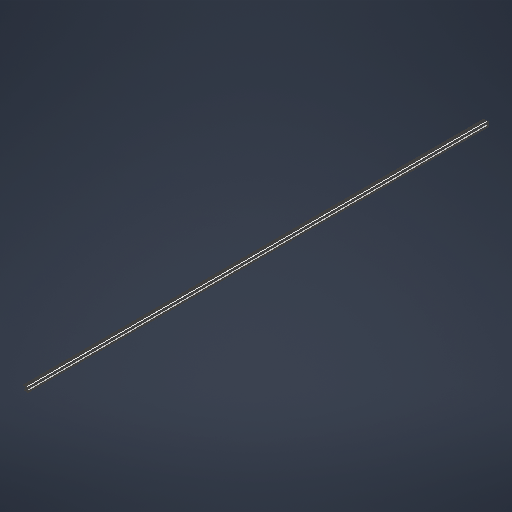
# Autodesk Inventor part: SP40-07 INVERSOR CENTRAL
Saved by Autodesk Inventor 2025 (Build 290162000, 162)
## iProperties
Created: 2026-01-24
Part Number: SP40-07 INVERSOR CENTRAL
Material: Aluminio
Document SubType Name: Modeling
Designer: ROLANDO
Density: 2.7 g/cm^3
Appearance: Satinado
Author: ROLANDO
Autodesk Inventor part; units mm, degrees
ref_plane "YZ Plane" through (0, 0, 0) normal (1, 0, 0) x (0, 1, 0)
ref_plane "XZ Plane" through (0, 0, 0) normal (0, 1, 0) x (-1, 0, 0)
ref_plane "XY Plane" through (0, 0, 0) normal (0, 0, 1) x (1, 0, 0)
sketch "Boceto1" plane through (0, 0, 0) normal (0, 0, 1) x (1, 0, 0)
  line L0 (8.6921, 12.0599) -> (8.6921, 49.4931)
  line L1 (8.6921, 10.6599) -> (-18.8079, 10.6599)
  line L2 (8.6921, 6.5599) -> (8.6921, 10.6599)
  line L3 (8.6921, 6.5599) -> (12.5921, 6.5599)
  line L4 (13.9921, 7.9599) -> (10.0921, 7.9599)
  line L5 (12.5921, 6.5599) -> (12.5921, 4.1599)
  line L6 (12.5921, 4.1599) -> (13.9921, 4.1599)
  line L7 (13.9921, 4.1599) -> (13.9921, 7.9599)
  line L8 (-13.0079, 12.0599) -> (-13.0079, 14.5599)
  line L9 (-13.0079, 14.5599) -> (-14.4079, 14.5599)
  line L10 (-14.4079, 14.5599) -> (-14.4079, 12.0599)
  line L11 (-8.6079, 12.0599) -> (-8.6079, 13.1599)
  line L12 (-8.6079, 14.5599) -> (-10.0079, 14.5599)
  line L13 (-10.0079, 14.5599) -> (-10.0079, 12.0599)
  line L14 (-7.2079, 14.1599) -> (-7.2079, 29.9599)
  line L15 (-8.6079, 29.5599) -> (-8.6079, 14.5599)
  line L16 (-17.4079, 12.0599) -> (-14.4079, 12.0599)
  line L17 (-17.4079, 12.0599) -> (-17.4079, 14.0599)
  line L18 (-18.8079, 12.9499) -> (-18.8079, 10.6599)
  line L19 (-17.4079, 14.0599) -> (-18.0102, 14.0599)
  line L20 (-18.0102, 14.0599) -> (-18.8079, 12.9499)
  line L21 (-8.6079, 29.5599) -> (-10.0079, 29.5599)
  line L22 (-10.0079, 29.5599) -> (-10.0079, 32.0599)
  line L23 (-8.6079, 33.4599) -> (-8.6079, 30.9599)
  line L24 (-18.8079, 29.4699) -> (-18.8079, 33.4599)
  line L25 (-14.4079, 32.0599) -> (-14.4079, 29.5599)
  line L26 (-14.4079, 29.5599) -> (-13.0079, 29.5599)
  line L27 (-13.0079, 29.5599) -> (-13.0079, 32.0599)
  line L28 (-10.0079, 32.0599) -> (-13.0079, 32.0599)
  line L29 (-14.4079, 32.0599) -> (-17.4079, 32.0599)
  line L30 (-17.4079, 32.0599) -> (-17.4079, 28.2599)
  line L31 (-17.4079, 28.2599) -> (-18.0191, 28.2599)
  line L32 (-13.0079, 33.4599) -> (-13.0079, 49.4999)
  line L33 (-14.4079, 49.4999) -> (-14.4079, 33.4599)
  line L34 (-18.8079, 33.4599) -> (-14.4079, 33.4599)
  line L35 (-13.0079, 33.4599) -> (-8.6079, 33.4599)
  line L36 (-13.0079, 49.4999) -> (-10.3179, 49.4999)
  line L37 (-10.3179, 49.4999) -> (-9.746, 50.1047)
  line L38 (-14.4079, 49.4999) -> (-17.0979, 49.4999)
  line L39 (-17.0979, 49.4999) -> (-17.5485, 49.9765)
  line L40 (-9.746, 50.1047) -> (8.6921, 49.4931)
  line L41 (-17.5485, 49.9765) -> (-27.9079, 49.669)
  line L42 (-27.9079, 49.669) -> (-27.9079, 45.6999)
  line L43 (-29.3079, 47.0999) -> (-29.3079, 49.4999)
  line L44 (-37.2079, 50.7936) -> (-37.2079, 45.6999)
  line L45 (-35.8079, 47.0999) -> (-35.8079, 49.4999)
  line L46 (-11.3879, 51.5599) -> (19.4921, 50.5356)
  line L47 (-11.3879, 51.5599) -> (-37.2079, 50.7936)
  line L48 (-8.6079, 30.9599) -> (-8.2079, 30.9599)
  line L49 (-8.6079, 13.1599) -> (-8.2079, 13.1599)
  line L50 (16.9921, 43.5999) -> (19.4921, 43.5999)
  line L51 (19.4921, 43.5999) -> (19.4921, 50.5356)
  line L52 (10.0921, 49.4466) -> (10.0921, 7.9599)
  line L53 (10.0921, 49.4466) -> (18.0921, 49.1812)
  line L54 (18.0921, 44.9999) -> (18.0921, 49.1812)
  line L55 (16.4921, 44.0999) -> (16.4921, 44.4999)
  line L56 (16.9921, 44.9999) -> (18.0921, 44.9999)
  line L57 (-13.0079, 12.0599) -> (-10.0079, 12.0599)
  line L58 (-8.6079, 12.0599) -> (8.6921, 12.0599)
  line L59 (-18.8079, 29.4699) -> (-18.0191, 28.2599)
  line L60 (-35.8079, 49.4999) -> (-29.3079, 49.4999)
  line L61 (-35.8079, 47.0999) -> (-34.5579, 47.0999)
  line L62 (-34.5579, 47.0999) -> (-34.5579, 46.3941)
  line L63 (-34.5579, 46.3941) -> (-35.5679, 45.6999)
  line L64 (-35.5679, 45.6999) -> (-37.2079, 45.6999)
  line L65 (-29.3079, 47.0999) -> (-30.5579, 47.0999)
  line L66 (-30.5579, 47.0999) -> (-30.5579, 46.3941)
  line L67 (-30.5579, 46.3941) -> (-29.5479, 45.6999)
  line L68 (-29.5479, 45.6999) -> (-27.9079, 45.6999)
  arc A0 (-7.2079, 29.9599) -> (-8.2079, 30.9599) centre (-8.2079, 29.9599) ccw
  arc A1 (-8.2079, 13.1599) -> (-7.2079, 14.1599) centre (-8.2079, 14.1599) ccw
  arc A2 (16.9921, 44.9999) -> (16.4921, 44.4999) centre (16.9921, 44.4999) ccw
  arc A3 (16.4921, 44.0999) -> (16.9921, 43.5999) centre (16.9921, 44.0999) ccw
  point P0 (0, 0)
  point P1 (-7.2079, 30.9599)
  point P2 (-7.2079, 13.1599)
  point P3 (16.4921, 43.5999)
  point P4 (16.4921, 44.9999)
  point P5 (-32.5579, 49.4999)
  dimension "d0" = 3.02
  dimension "d1" = 24.5
  dimension "d2" = 1.4
  dimension "d3" = 1.4
  dimension "d4" = 1.4
  dimension "d5" = 1.4
  dimension "d7" = 1.4
  dimension "d8" = 1.4
  dimension "d9" = 1.4
  dimension "d10" = 1.4
  dimension "d11" = 1.4
  dimension "d12" = 1.4
  dimension "d13" = 1.4
  dimension "d14" = 1.4
  dimension "d15" = 1.4
  dimension "d16" = 1.4
  dimension "d17" = 1.4
  dimension "d23" = 1.4
  dimension "d26" = 3
  dimension "d27" = 39.44
  dimension "d31" = 7.9
  dimension "d32" = 2.4
  dimension "d34" = 2.5
  dimension "d35" = 2.5
  dimension "d36" = 3
  dimension "d37" = 3
  dimension "d38" = 3
  dimension "d39" = 3
  dimension "d42" = 4.09
  dimension "d43" = 2.69
  dimension "d44" = 15
  dimension "d45" = 20
  dimension "d47" = 2
  dimension "d48" = 1.11
  dimension "d51" = 1.21
  dimension "d52" = 35.7
  dimension "d53" = 33.1
  dimension "d55" = 32.8
  dimension "d56" = 14.2
  dimension "d58" = 15.9
  dimension "d65" = 1.4
  dimension "d68" = 46.6
  dimension "d69" = 46.6
  dimension "d70" = 2.06
  dimension "d73" = 91.7
  dimension "d74" = 91.9
  dimension "d77" = 1.4
  dimension "d84" = 1.4
  dimension "d87" = 6.5
  dimension "d88" = 9.3
  dimension "d89" = 1.4
  dimension "d90" = 1.4
  dimension "d91" = 3.25
  dimension "d92" = 1.4
  dimension "d93" = 2
  dimension "d96" = 3.01
  dimension "d97" = 6.02
  dimension "d99" = 34.5
  dimension "d100" = 111
  dimension "d102" = 2.4
  dimension "d104" = 1.4
  dimension "d105" = 22.8
  dimension "d106" = 4
  dimension "d107" = 0.7058
  constraints: 138 end point, 22 parallel, 20 collinear, 14 horizontal, 9 perpendicular, 9 point on line, 8 point on circle, 8 tangent, 6 vertical, 4 centre point, 2 equal radius, 1 coincident, 1 midpoint, 2 other
  measures "d0" distance from line of L33 L46.start
  measures "d1" distance between parallel lines of L52 L33
  measures "d2" distance between parallel lines of L0 L52
  measures "d3" distance between parallel lines of L33 L32
  measures "d4" distance between parallel lines of L51 L54
  measures "d5" distance between parallel lines of L56 L50
  measures "d7" distance between parallel lines of L15 L14
  measures "d8" distance between parallel lines of L4 L3
  measures "d9" distance between parallel lines of L7 L5
  measures "d10" distance between parallel lines of L58 L1
  measures "d11" distance between parallel lines of L8 L10
  measures "d12" distance between parallel lines of L17 L18
  measures "d13" distance between parallel lines of L34 L29
  measures "d14" distance between parallel lines of L25 L27
  measures "d15" distance between parallel lines of L23 L22
  measures "d16" distance between parallel lines of L21 L48
  measures "d17" distance between parallel lines of L49 L12
  measures "d23" distance between parallel lines of L24 L30
  measures "d26" distance between parallel lines of L51 L55
  measures "d27" distance between parallel lines of L6 L50
  measures "d31" distance between parallel lines of L6 L58
  measures "d32" distance between parallel lines of L3 L6
  measures "d34" distance between parallel lines of L12 L58
  measures "d35" distance between parallel lines of L21 L28
  measures "d36" distance between parallel lines of L8 L13
  measures "d37" distance between parallel lines of L27 L22
  measures "d38" distance between parallel lines of L17 L10
  measures "d39" distance between parallel lines of L30 L25
  measures "d42" distance from line of L33 L36.end
  measures "d43" distance from line of L33 L38.end
  measures "d44" distance between parallel lines of L9 L26
  measures "d45" distance between parallel lines of L16 L29
  measures "d47" distance between parallel lines of L19 L16
  measures "d48" vertical distance of L19.end L18.start
  measures "d51" vertical distance of L31.end L24.start
  measures "d52" angle of L18 L20
  measures "d53" angle of L24 L59
  measures "d55" distance between parallel lines of L7 L18
  measures "d56" distance between parallel lines of L19 L31
  measures "d58" distance between parallel lines of L0 L14
  measures "d65" distance between parallel lines of L13 L15
  measures "d68" angle of L38 L39
  measures "d69" angle of L36 L37
  measures "d70" distance from line of L46.start L36
  measures "d73" angle of L47 L44
  measures "d74" angle of L51 L46
  measures "d77" distance between parallel lines of L46 L53
  measures "d84" distance between parallel lines of L47 L41
  measures "d87" distance between parallel lines of L43 L45
  measures "d88" distance between parallel lines of L42 L44
  measures "d89" distance between parallel lines of L43 L42
  measures "d90" distance between parallel lines of L44 L45
  measures "d91" distance from line of L43 point (-32.558, 49.5)
  measures "d92" distance between parallel lines of L61 L64
  measures "d93" distance from line of L66 point (-32.558, 49.5)
  measures "d96" horizontal distance of point (-32.558, 49.5) L63.end
  measures "d97" distance of L67.end L63.end
  measures "d99" angle of L64 L63
  measures "d100" angle of L67 L63
  measures "d102" distance between parallel lines of L60 L61
  measures "d104" distance between parallel lines of L46 L40
  measures "d105" distance between parallel lines of L44 L33
  measures "d106" distance of L62.end L66.end
  measures "d107" distance of L61.end L62.end
extrude "Extrusión1" add sketch "Boceto1" against normal blind 5000
